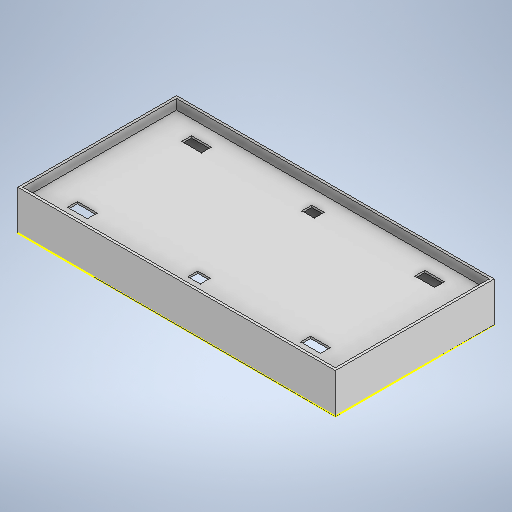
# Autodesk Inventor part: led_spectrum_frame
Saved by Autodesk Inventor 2025.2 (Build 292293000, 293)
## iProperties
Created: 2026-07-12
Part Number: led_spectrum_frame
Material: Generic
Document SubType Name: Modeling
Designer: Emlin
Density: 1 g/cm^3
Appearance: Default
Author: Emlin
Autodesk Inventor part; units mm, degrees
note: some values were not read from the file. Chosen so that the rebuilt part matches the saved one: second side of "Extrusion1".
ref_plane "YZ Plane" through (0, 0, 0) normal (1, 0, 0) x (0, 1, 0)
ref_plane "XZ Plane" through (0, 0, 0) normal (0, 1, 0) x (-1, 0, 0)
ref_plane "XY Plane" through (0, 0, 0) normal (0, 0, 1) x (1, 0, 0)
sketch "Sketch1" plane through (0, 0, 0) normal (0, 1, 0) x (-1, 0, 0)
  line L0 (0, 0) -> (-320, 0)
  line L1 (-320, 0) -> (-320, -160)
  line L2 (-320, -160) -> (0, -160)
  line L3 (0, -160) -> (0, 0)
  line L4 (-2.5, -157.5) -> (-317.5, -157.5)
  line L5 (-317.5, -157.5) -> (-317.5, -2.5)
  line L6 (-317.5, -2.5) -> (-2.5, -2.5)
  line L7 (-2.5, -2.5) -> (-2.5, -157.5)
  line L8 (-32.5, -142.5) -> (-52.5, -142.5)
  line L9 (-52.5, -142.5) -> (-52.5, -132.5)
  line L10 (-52.5, -132.5) -> (-32.5, -132.5)
  line L11 (-32.5, -132.5) -> (-32.5, -142.5)
  line L12 (-287.5, -142.5) -> (-267.5, -142.5)
  line L13 (-267.5, -142.5) -> (-267.5, -132.5)
  line L14 (-267.5, -132.5) -> (-287.5, -132.5)
  line L15 (-287.5, -132.5) -> (-287.5, -142.5)
  line L16 (-166.25, -142.5) -> (-153.75, -142.5)
  line L17 (-153.75, -142.5) -> (-153.75, -132.5)
  line L18 (-153.75, -132.5) -> (-166.25, -132.5)
  line L19 (-166.25, -132.5) -> (-166.25, -142.5)
  line L20 (-2.5, -80) -> (-317.5, -80)
  line L21 (-32.5, -17.5) -> (-52.5, -17.5)
  line L22 (-52.5, -17.5) -> (-52.5, -27.5)
  line L23 (-52.5, -27.5) -> (-32.5, -27.5)
  line L24 (-32.5, -27.5) -> (-32.5, -17.5)
  line L25 (-287.5, -17.5) -> (-267.5, -17.5)
  line L26 (-267.5, -17.5) -> (-267.5, -27.5)
  line L27 (-267.5, -27.5) -> (-287.5, -27.5)
  line L28 (-287.5, -27.5) -> (-287.5, -17.5)
  line L29 (-166.25, -17.5) -> (-153.75, -17.5)
  line L30 (-153.75, -17.5) -> (-153.75, -27.5)
  line L31 (-153.75, -27.5) -> (-166.25, -27.5)
  line L32 (-166.25, -27.5) -> (-166.25, -17.5)
  point P0 (-32.5, -137.5)
  point P1 (-42.5, -142.5)
  point P2 (-277.5, -142.5)
  point P3 (-287.5, -137.5)
  point P4 (-52.5, -137.5)
  point P5 (-267.5, -137.5)
  point P6 (-160, -142.5)
  point P7 (-32.5, -22.5)
  point P8 (-42.5, -17.5)
  point P9 (-277.5, -17.5)
  point P10 (-287.5, -22.5)
  point P11 (-52.5, -22.5)
  point P12 (-267.5, -22.5)
  point P13 (-160, -17.5)
  dimension "d0" = 320
  dimension "d1" = 160
  dimension "d2" = 2.5
  dimension "d7" = 30
  dimension "d8" = 15
  dimension "d9" = 20
  dimension "d10" = 10
  dimension "d11" = 20
  dimension "d12" = 10
  dimension "d13" = 15
  dimension "d14" = 30
  dimension "d16" = 215
  dimension "d18" = 10
  dimension "d19" = 12.5
  dimension "d23" = 160
  dimension "d25" = 15
  constraints: 66 end point, 19 symmetric about line, 10 parallel, 9 midpoint, 5 perpendicular, 4 horizontal, 3 other
  measures "d0" distance of L1.end L2.end
  measures "d1" distance of L0.end L1.end
  measures "d2" distance between parallel lines of L2 L4
  measures "d7" distance from line of L7 point (-32.5, -137.5)
  measures "d8" distance from line of L4 point (-42.5, -142.5)
  measures "d9" distance of L9.end L10.end
  measures "d10" distance of L8.end L9.end
  measures "d11" distance of L13.end L14.end
  measures "d12" distance of L12.end L13.end
  measures "d13" distance from line of L4 point (-277.5, -142.5)
  measures "d14" distance from line of L5 point (-287.5, -137.5)
  measures "d16" distance of point (-52.5, -137.5) point (-267.5, -137.5)
  measures "d18" distance of L16.end L17.end
  measures "d19" distance of L16.start L16.end
  measures "d23" distance from line of L3 point (-160, -142.5)
  measures "d25" distance between parallel lines of L4 L16
extrude "Extrusion1" add sketch "Sketch1" along normal blind 2 contours L3 L2 L1 L0 | L4 L5 L20 L7 | L20 L5 L6 L7
sketch "Sketch2" plane through (0, 2, 0) normal (0, 1, 0) x (1, 0, 0)
  line L0 (320, 0) -> (320, 160) projected
  line L1 (320, 160) -> (0, 160) projected
  line L2 (0, 160) -> (0, 0) projected
  line L3 (0, 0) -> (320, 0) projected
  line L4 (32.5, 142.5) -> (52.5, 142.5) projected
  line L5 (52.5, 142.5) -> (52.5, 132.5) projected
  line L6 (52.5, 132.5) -> (32.5, 132.5) projected
  line L7 (32.5, 132.5) -> (32.5, 142.5) projected
  line L8 (287.5, 142.5) -> (287.5, 132.5) projected
  line L9 (287.5, 132.5) -> (267.5, 132.5) projected
  line L10 (267.5, 132.5) -> (267.5, 142.5) projected
  line L11 (267.5, 142.5) -> (287.5, 142.5) projected
  line L12 (166.25, 142.5) -> (166.25, 132.5) projected
  line L13 (166.25, 132.5) -> (153.75, 132.5) projected
  line L14 (153.75, 132.5) -> (153.75, 142.5) projected
  line L15 (153.75, 142.5) -> (166.25, 142.5) projected
  line L16 (52.5, 17.5) -> (32.5, 17.5) projected
  line L17 (32.5, 17.5) -> (32.5, 27.5) projected
  line L18 (32.5, 27.5) -> (52.5, 27.5) projected
  line L19 (52.5, 27.5) -> (52.5, 17.5) projected
  line L20 (267.5, 17.5) -> (267.5, 27.5) projected
  line L21 (267.5, 27.5) -> (287.5, 27.5) projected
  line L22 (287.5, 27.5) -> (287.5, 17.5) projected
  line L23 (287.5, 17.5) -> (267.5, 17.5) projected
  line L24 (166.25, 27.5) -> (166.25, 17.5) projected
  line L25 (166.25, 17.5) -> (153.75, 17.5) projected
  line L26 (153.75, 17.5) -> (153.75, 27.5) projected
  line L27 (153.75, 27.5) -> (166.25, 27.5) projected
  line L28 (2.5, 2.5) -> (2.5, 157.5)
  line L29 (2.5, 157.5) -> (317.5, 157.5)
  line L30 (317.5, 157.5) -> (317.5, 2.5)
  line L31 (317.5, 2.5) -> (2.5, 2.5)
  dimension "d26" = 2.5
  constraints: 8 end point, 3 other
  measures "d26" distance between parallel lines of L2 L28
extrude "Extrusion2" add sketch "Sketch2" along normal blind 10 and the other way blind 30 contours L3 L2 L1 L0
sketch "Sketch3" plane through (0, -28, 0) normal (0, -1, 0) x (1, 0, 0)
  line L0 (0, 0) -> (0, -160) projected
  line L1 (0, -160) -> (320, -160) projected
  line L2 (320, -160) -> (320, 0) projected
  line L3 (320, 0) -> (0, 0) projected
body "Solid1"
